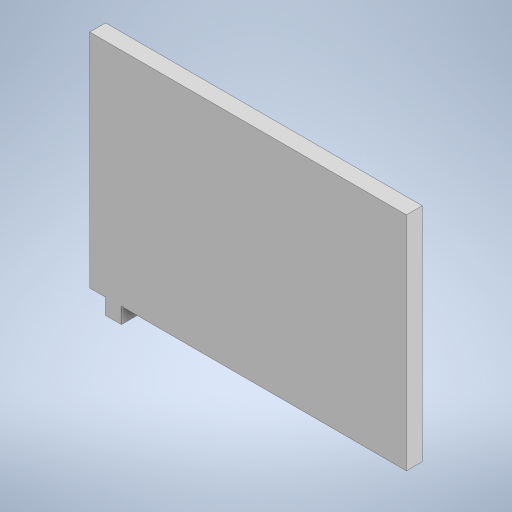
# Autodesk Inventor part: backside
Saved by Autodesk Inventor 2024 (Build 280153000, 153)
## iProperties
Created: 2024-04-15
Part Number: backside
Material: Generic
Document SubType Name: Modeling
Designer: srika
Density: 1 g/cm^3
Appearance: Default
Author: srika
Autodesk Inventor part; units mm, degrees
ref_plane "YZ Plane" through (0, 0, 0) normal (1, 0, 0) x (0, 1, 0)
ref_plane "XZ Plane" through (0, 0, 0) normal (0, 1, 0) x (-1, 0, 0)
ref_plane "XY Plane" through (0, 0, 0) normal (0, 0, 1) x (1, 0, 0)
sketch "Sketch2" plane through (0, 0, 0) normal (0, 0, 1) x (1, 0, 0)
  line L0 (0, 0) -> (5, 0)
  line L1 (5, 0) -> (5, 5)
  line L2 (5, 5) -> (0, 5)
  line L3 (0, 5) -> (0, 0)
  line L4 (5, 5) -> (105, 5)
  line L5 (5, 55) -> (5, 5)
  line L6 (15, 5) -> (10, 5)
  line L7 (10, 0) -> (15, 0)
  line L8 (15, 0) -> (15, 5)
  line L9 (10, 5) -> (10, 0)
  line L10 (25, 5) -> (20, 5)
  line L11 (20, 0) -> (25, 0)
  line L12 (25, 0) -> (25, 5)
  line L13 (20, 5) -> (20, 0)
  line L14 (35, 5) -> (30, 5)
  line L15 (30, 0) -> (35, 0)
  line L16 (35, 0) -> (35, 5)
  line L17 (30, 5) -> (30, 0)
  line L18 (45, 5) -> (40, 5)
  line L19 (40, 0) -> (45, 0)
  line L20 (45, 0) -> (45, 5)
  line L21 (40, 5) -> (40, 0)
  line L22 (55, 5) -> (50, 5)
  line L23 (50, 0) -> (55, 0)
  line L24 (55, 0) -> (55, 5)
  line L25 (50, 5) -> (50, 0)
  line L26 (65, 5) -> (60, 5)
  line L27 (60, 0) -> (65, 0)
  line L28 (65, 0) -> (65, 5)
  line L29 (60, 5) -> (60, 0)
  line L30 (75, 5) -> (70, 5)
  line L31 (70, 0) -> (75, 0)
  line L32 (75, 0) -> (75, 5)
  line L33 (70, 5) -> (70, 0)
  line L34 (85, 5) -> (80, 5)
  line L35 (80, 0) -> (85, 0)
  line L36 (85, 0) -> (85, 5)
  line L37 (80, 5) -> (80, 0)
  line L38 (95, 5) -> (90, 5)
  line L39 (90, 0) -> (95, 0)
  line L40 (95, 0) -> (95, 5)
  line L41 (90, 5) -> (90, 0)
  line L42 (105, 5) -> (100, 5)
  line L43 (100, 0) -> (105, 0)
  line L44 (105, 0) -> (105, 5)
  line L45 (100, 5) -> (100, 0)
  circle A0 centre (12.3298, 65) radius 3.5
  line L46 (6.3298, 40) -> (18.3298, 40)
  line L47 (18.3298, 40) -> (18.3298, 70)
  line L48 (18.3298, 70) -> (6.3298, 70)
  line L49 (6.3298, 70) -> (6.3298, 40)
  line L50 (6.3298, 40) -> (18.3298, 70) construction
  line L51 (18.3298, 40) -> (6.3298, 70) construction
  line L52 (19, 40) -> (31, 40)
  circle A1 centre (25, 65) radius 3.5
  line L53 (19, 70) -> (19, 40)
  line L54 (31, 40) -> (31, 70)
  line L55 (19, 40) -> (31, 70) construction
  line L56 (31, 40) -> (19, 70) construction
  line L57 (31, 70) -> (19, 70)
  line L58 (31.5, 40) -> (43.5, 40)
  circle A2 centre (37.5, 65) radius 3.5
  line L59 (31.5, 70) -> (31.5, 40)
  line L60 (43.5, 40) -> (43.5, 70)
  line L61 (31.5, 40) -> (43.5, 70) construction
  line L62 (43.5, 40) -> (31.5, 70) construction
  line L63 (43.5, 70) -> (31.5, 70)
  line L64 (44.1702, 70) -> (44.1702, 40)
  line L65 (56.1702, 40) -> (56.1702, 70)
  line L66 (56.1702, 40) -> (44.1702, 70) construction
  line L67 (44.1702, 40) -> (56.1702, 70) construction
  line L68 (56.1702, 70) -> (44.1702, 70)
  circle A3 centre (50.1702, 65) radius 3.5
  line L69 (44.1702, 40) -> (56.1702, 40)
  line L70 (57.3642, 39.8119) -> (69.3642, 39.8119)
  line L71 (57.3642, 69.8119) -> (57.3642, 39.8119)
  line L72 (69.3642, 69.8119) -> (57.3642, 69.8119)
  line L73 (57.3642, 39.8119) -> (69.3642, 69.8119) construction
  line L74 (69.3642, 39.8119) -> (57.3642, 69.8119) construction
  line L75 (69.3642, 39.8119) -> (69.3642, 69.8119)
  circle A4 centre (63.3642, 64.8119) radius 3.5
  line L76 (75, 40) -> (100, 40)
  line L77 (100, 40) -> (100, 70)
  line L78 (100, 70) -> (75, 70)
  line L79 (75, 70) -> (75, 40)
  line L80 (75, 40) -> (100, 70) construction
  line L81 (100, 40) -> (75, 70) construction
  line L82 (82.75, 63.25) -> (92.25, 63.25)
  line L83 (92.25, 63.25) -> (92.25, 66.75)
  line L84 (92.25, 66.75) -> (82.75, 66.75)
  line L85 (82.75, 66.75) -> (82.75, 63.25)
  line L86 (82.75, 63.25) -> (92.25, 66.75) construction
  line L87 (92.25, 63.25) -> (82.75, 66.75) construction
  line L88 (5, 75) -> (105, 75)
  line L89 (105, 75) -> (105, 5)
  line L90 (5, 75) -> (5, 55)
  line L91 (105, 80) -> (110, 80)
  line L92 (110, 80) -> (110, 75)
  line L93 (110, 75) -> (105, 75)
  line L94 (105, 75) -> (105, 80)
  line L95 (105, 65) -> (105, 70)
  line L96 (110, 65) -> (105, 65)
  line L97 (110, 70) -> (110, 65)
  line L98 (105, 70) -> (110, 70)
  line L99 (105, 55) -> (105, 60)
  line L100 (110, 55) -> (105, 55)
  line L101 (110, 60) -> (110, 55)
  line L102 (105, 60) -> (110, 60)
  line L103 (105, 45) -> (105, 50)
  line L104 (110, 45) -> (105, 45)
  line L105 (110, 50) -> (110, 45)
  line L106 (105, 50) -> (110, 50)
  line L107 (105, 35) -> (105, 40)
  line L108 (110, 35) -> (105, 35)
  line L109 (110, 40) -> (110, 35)
  line L110 (105, 40) -> (110, 40)
  line L111 (105, 25) -> (105, 30)
  line L112 (110, 25) -> (105, 25)
  line L113 (110, 30) -> (110, 25)
  line L114 (105, 30) -> (110, 30)
  line L115 (105, 15) -> (105, 20)
  line L116 (110, 15) -> (105, 15)
  line L117 (110, 20) -> (110, 15)
  line L118 (105, 20) -> (110, 20)
  line L119 (105, 5) -> (105, 10)
  line L120 (110, 5) -> (105, 5)
  line L121 (110, 10) -> (110, 5)
  line L122 (105, 10) -> (110, 10)
  line L123 (95, 80) -> (100, 80)
  line L124 (100, 80) -> (100, 75)
  line L125 (95, 75) -> (95, 80)
  line L126 (100, 75) -> (95, 75)
  line L127 (85, 80) -> (90, 80)
  line L128 (90, 80) -> (90, 75)
  line L129 (85, 75) -> (85, 80)
  line L130 (90, 75) -> (85, 75)
  line L131 (75, 80) -> (80, 80)
  line L132 (80, 80) -> (80, 75)
  line L133 (75, 75) -> (75, 80)
  line L134 (80, 75) -> (75, 75)
  line L135 (65, 80) -> (70, 80)
  line L136 (70, 80) -> (70, 75)
  line L137 (65, 75) -> (65, 80)
  line L138 (70, 75) -> (65, 75)
  line L139 (55, 80) -> (60, 80)
  line L140 (60, 80) -> (60, 75)
  line L141 (55, 75) -> (55, 80)
  line L142 (60, 75) -> (55, 75)
  line L143 (45, 80) -> (50, 80)
  line L144 (50, 80) -> (50, 75)
  line L145 (45, 75) -> (45, 80)
  line L146 (50, 75) -> (45, 75)
  line L147 (35, 80) -> (40, 80)
  line L148 (40, 80) -> (40, 75)
  line L149 (35, 75) -> (35, 80)
  line L150 (40, 75) -> (35, 75)
  line L151 (25, 80) -> (30, 80)
  line L152 (30, 80) -> (30, 75)
  line L153 (25, 75) -> (25, 80)
  line L154 (30, 75) -> (25, 75)
  line L155 (15, 80) -> (20, 80)
  line L156 (20, 80) -> (20, 75)
  line L157 (15, 75) -> (15, 80)
  line L158 (20, 75) -> (15, 75)
  line L159 (5, 80) -> (10, 80)
  line L160 (10, 80) -> (10, 75)
  line L161 (5, 75) -> (5, 80)
  line L162 (10, 75) -> (5, 75)
  line L163 (0, 10) -> (5, 10)
  line L164 (5, 10) -> (5, 15)
  line L165 (5, 15) -> (0, 15)
  line L166 (0, 15) -> (0, 10)
  line L167 (0, 20) -> (5, 20)
  line L168 (5, 20) -> (5, 25)
  line L169 (5, 25) -> (0, 25)
  line L170 (0, 25) -> (0, 20)
  line L171 (0, 30) -> (5, 30)
  line L172 (5, 30) -> (5, 35)
  line L173 (5, 35) -> (0, 35)
  line L174 (0, 35) -> (0, 30)
  line L175 (0, 40) -> (5, 40)
  line L176 (5, 40) -> (5, 45)
  line L177 (5, 45) -> (0, 45)
  line L178 (0, 45) -> (0, 40)
  line L179 (0, 50) -> (5, 50)
  line L180 (5, 50) -> (5, 55)
  line L181 (5, 55) -> (0, 55)
  line L182 (0, 55) -> (0, 50)
  line L183 (0, 60) -> (5, 60)
  line L184 (5, 60) -> (5, 65)
  line L185 (5, 65) -> (0, 65)
  line L186 (0, 65) -> (0, 60)
  line L187 (0, 70) -> (5, 70)
  line L188 (5, 70) -> (5, 75)
  line L189 (5, 75) -> (0, 75)
  line L190 (0, 75) -> (0, 70)
  line L191 (100, 10) -> (25, 10)
  line L192 (25, 10) -> (25, 35)
  line L193 (25, 35) -> (100, 35)
  line L194 (100, 35) -> (100, 10)
  point P0 (87.5, 55)
  point P1 (87.5, 65)
  dimension "d0" = 5
  dimension "d1" = 5
  dimension "d29" = 10
  dimension "d37" = 7
  dimension "d38" = 12
  dimension "d39" = 30
  dimension "d51" = 7
  dimension "d52" = 12
  dimension "d53" = 30
  dimension "d54" = 7
  dimension "d55" = 12
  dimension "d56" = 30
  dimension "d57" = 7
  dimension "d58" = 12
  dimension "d59" = 30
  dimension "d60" = 7
  dimension "d61" = 12
  dimension "d62" = 30
  dimension "d63" = 25
  dimension "d64" = 30
  dimension "d65" = 9.5
  dimension "d66" = 3.5
  dimension "d71" = 10
  dimension "d78" = 10
  dimension "d85" = 10
  constraints: 388 end point, 40 horizontal alignment, 40 parallel, 21 collinear, 12 horizontal, 11 perpendicular, 5 centre point, 4 midpoint, 2 vertical, 1 point on line, 202 other
  measures "d0" distance of L2.end L1.end
  measures "d1" distance of L1.end L0.end
  measures "d29" distance of L2.end L6.end
  measures "d37" diameter of A0
  measures "d38" distance of L49.start L47.end
  measures "d39" distance of L47.end L46.end
  measures "d51" diameter of A1
  measures "d52" distance of L53.start L54.end
  measures "d53" distance of L54.end L54.start
  measures "d54" diameter of A2
  measures "d55" distance of L63.end L60.end
  measures "d56" distance of L60.end L60.start
  measures "d57" diameter of A3
  measures "d58" distance of L64.start L68.start
  measures "d59" distance of L68.start L69.end
  measures "d60" diameter of A4
  measures "d61" distance of L71.start L72.start
  measures "d62" distance of L72.start L70.end
  measures "d63" distance of L78.end L77.end
  measures "d64" distance of L77.end L76.end
  measures "d65" distance of L84.end L83.end
  measures "d66" distance of L83.end L82.end
  measures "d71" distance of L88.end point (105, 65)
  measures "d78" distance of L91.start L123.start
  measures "d85" distance of L0.start L163.start
extrude "Extrusion1" add sketch "Sketch2" along normal blind 5 contours L5 L90 L88 L89 L4 | L4 L8 L7 L9 | A0 | L49 L48 L47 L46 | L53 L57 L54 L52 | A1 | L59 L63 L60 L58 | A2 | L68 L65 L69 L64 | A3 | L71 L72 L75 L70 | A4 | L79 L78 L77 L76 | L85 L84 L83 L82 | L191 L192 L193 L194
body "Solid1"
